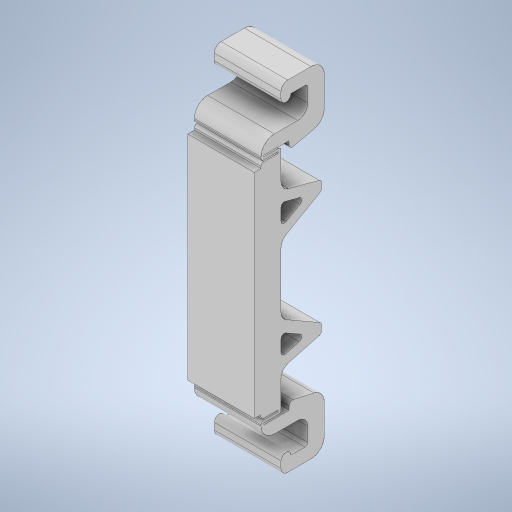
# Autodesk Inventor part: DIN-rail-mount
Saved by Autodesk Inventor 2023 (Build 270158030, 158C)
## iProperties
Created: 2024-03-20
Part Number: DIN-rail-mount
Material: Generic
Document SubType Name: Modeling
Designer: Imogen Heard
Density: 1 g/cm^3
Appearance: Default
Author: Imogen Heard
Autodesk Inventor part; units mm, degrees
ref_plane "YZ Plane" through (0, 0, 0) normal (1, 0, 0) x (0, 1, 0)
ref_plane "XZ Plane" through (0, 0, 0) normal (0, 1, 0) x (-1, 0, 0)
ref_plane "XY Plane" through (0, 0, 0) normal (0, 0, 1) x (1, 0, 0)
sketch "DIN-rail-clip-generic-V1.0" plane through (0, 0, 0) normal (0, 0, 1) x (1, 0, 0)
  line L0 (0, 40.9467) -> (3, 40.9467)
  line L1 (3, 40.9467) -> (3, 17.5)
  line L2 (3, 17.5) -> (0, 17.5)
  line L3 (0, 17.5) -> (0, 40.9467)
  line L4 (0, 35.1) -> (-0.3528, 35.269) construction
  line L5 (-0.3528, 35.269) -> (-1.1784, 35.269) construction
  line L6 (-1.1784, 35.269) -> (-1.277, 34.6657) construction
  line L7 (-1.277, 34.6657) -> (-0.9372, 34.5565) construction
  line L8 (-0.9372, 34.5565) -> (-2.5363, 34.2808) construction
  line L9 (-2.5363, 34.2808) -> (-3.3649, 34.5884) construction
  line L10 (-3.3649, 34.5884) -> (-4.7205, 35.8697) construction
  line L11 (-4.7205, 35.8697) -> (-5.1321, 37.4532) construction
  line L12 (-5.1321, 37.4532) -> (-5.1209, 40.8876) construction
  line L13 (-5.1209, 40.8876) -> (-4.7, 42.1113) construction
  line L14 (-4.7, 42.1113) -> (-3.9, 43.3113) construction
  line L15 (-3.9, 43.3113) -> (-2.1, 44.1113) construction
  line L16 (-2.1, 44.1113) -> (0, 43.5467) construction
  line L17 (0, 43.5467) -> (0.1036, 42.9467) construction
  line L18 (0.1036, 42.9467) -> (-0.2, 41.9467) construction
  line L19 (-0.2, 41.9467) -> (-1.1, 42.4004) construction
  line L20 (-1.1, 42.4004) -> (-2.3, 42.4379) construction
  spline S0 degree 4 poles (0, 35.1) (-0.3528, 35.269) (-1.1784, 35.269) (-1.277, 34.6657) (-0.9372, 34.5565) (-2.5363, 34.2808) (-3.3649, 34.5884) (-4.7205, 35.8697) (-5.1321, 37.4532) (-5.1209, 40.8876) (-4.7, 42.1113) (-3.9, 43.3113) (-2.1, 44.1113) (0, 43.5467) (0.1036, 42.9467) (-0.2, 41.9467) (-1.1, 42.4004) (-2.3, 42.4379) (-2.2829, 41.0379) (-1.7552, 41.1368) (0, 40.9467) knots 1 1 1 1 1 2 3 4 5 6 7 8 9 10 11 12 13 14 15 16 17 17.993985 17.993985 17.993985 17.993985 17.993985
  line L21 (0, 35.8905) -> (-0.7907, 36.0877) construction
  line L22 (-0.7907, 36.0877) -> (-1.1784, 36.0877) construction
  line L23 (-1.1784, 36.0877) -> (-2.2779, 36.5342) construction
  line L24 (-2.2779, 36.5342) -> (-2.7458, 36.6343) construction
  line L25 (-2.7458, 36.6343) -> (-3.471, 38.3527) construction
  line L26 (-3.471, 38.3527) -> (-2.7458, 40.1075) construction
  spline S1 degree 4 poles (0, 35.8905) (-0.7907, 36.0877) (-1.1784, 36.0877) (-2.2779, 36.5342) (-2.7458, 36.6343) (-3.471, 38.3527) (-2.7458, 40.1075) (-2.4429, 40.6075) (-0.7055, 40.4056) (0, 40.2568) knots 1 1 1 1 1 2 3 4 5 6 6.977977 6.977977 6.977977 6.977977 6.977977
  line L27 (-2.3, 42.4379) -> (-2.2829, 41.0379) construction
  line L28 (-2.2829, 41.0379) -> (-1.7552, 41.1368) construction
  line L29 (-1.7552, 41.1368) -> (0, 40.9467) construction
  line L30 (-2.7458, 40.1075) -> (-2.4429, 40.6075) construction
  line L31 (-2.4429, 40.6075) -> (-0.7055, 40.4056) construction
  line L32 (-0.7055, 40.4056) -> (0, 40.2568) construction
  line L33 (0, 36.6343) -> (-1.1784, 36.9758) construction
  line L34 (-1.1784, 36.9758) -> (-2.2101, 37.6402) construction
  line L35 (-2.2101, 37.6402) -> (-2.1452, 38.3006) construction
  line L36 (-2.1452, 38.3006) -> (-1.8076, 39.3817) construction
  line L37 (-1.8076, 39.3817) -> (-0.8778, 39.5886) construction
  line L38 (-0.8778, 39.5886) -> (0, 39.5886) construction
  spline S2 degree 4 poles (0, 36.6343) (-1.1784, 36.9758) (-2.2101, 37.6402) (-2.1452, 38.3006) (-1.8076, 39.3817) (-0.8778, 39.5886) (0, 39.5886) knots 1 1 1 1 1 2 3 4 4 4 4 4
  line L39 (-0.5144, 23.8721) -> (0, 22.0778) construction
  spline S3 degree 4 poles (0, 28.5164) (-0.0002, 28.5161) (-0.1764, 28.1682) (-0.5144, 27.8581) (-1.1668, 26.9412) (-3.3762, 27.1074) (-5.9868, 27.5396) (-6.4206, 26.5054) (-5.8606, 24.9054) (-2.8606, 24.6412) (-1.4606, 24.4656) (-0.5144, 23.8721) (0, 22.0778) knots 1 1 1 1 1 1.050464 1.110527 1.512977 1.739488 1.83789 2 2.236311 2.876473 3 3 3 3 3
  line L40 (-1.4606, 24.4656) -> (-0.5144, 23.8721) construction
  line L41 (-3.3762, 27.1074) -> (-5.9868, 27.5396) construction
  line L42 (-5.9868, 27.5396) -> (-6.4206, 26.5054) construction
  line L43 (-6.4206, 26.5054) -> (-5.8606, 24.9054) construction
  line L44 (-5.8606, 24.9054) -> (-2.8606, 24.6412) construction
  line L45 (-2.8606, 24.6412) -> (-1.4606, 24.4656) construction
  line L46 (0, 28.5164) -> (-0.1764, 28.1682) construction
  line L47 (-0.1764, 28.1682) -> (-0.5144, 27.8581) construction
  line L48 (-0.5144, 27.8581) -> (-1.1668, 26.9412) construction
  line L49 (-1.1668, 26.9412) -> (-3.3762, 27.1074) construction
  circle A0 centre (1, 40.9467) radius 0.7
  point P0 (0, 17.5)
  point P1 (-0.5, 35)
  point P2 (-1, 33.6)
  dimension "d63" = 3
  dimension "d68" = 23.4467
  dimension "d71" = 0.9373
  dimension "d73" = 0.269
  dimension "d74" = 0.3528
  dimension "d79" = 1.5363
  dimension "d85" = 0.7905
  dimension "d87" = 1.1784
  dimension "d88" = 0.7907
  dimension "d89" = 1.5835
  dimension "d90" = 5.1321
  dimension "d92" = 2.2779
  dimension "d93" = 2.7458
  dimension "d95" = 1.7184
  dimension "d96" = 0.7252
  dimension "d97" = 3.4344
  dimension "d99" = 1.2236
  dimension "d100" = 0.4209
  dimension "d101" = 1.2
  dimension "d102" = 0.8
  dimension "d103" = 1.8
  dimension "d104" = 0.8
  dimension "d105" = 2.6
  dimension "d106" = 0.1036
  dimension "d107" = 2
  dimension "d108" = 0.2
  dimension "d109" = 1
  dimension "d110" = 0.9
  dimension "d111" = 0.4536
  dimension "d112" = 1.2
  dimension "d113" = 1.4
  dimension "d114" = 0.0375
  dimension "d115" = 0.0171
  dimension "d116" = 0.5278
  dimension "d117" = 0.0989
  dimension "d118" = 0.69
  dimension "d119" = 0.6682
  dimension "d120" = 0.7055
  dimension "d121" = 0.5412
  dimension "d122" = 1.7374
  dimension "d123" = 0.2019
  dimension "d124" = 0.5
  dimension "d125" = 0.3029
  dimension "d126" = 1.1784
  dimension "d127" = 3.9709
  dimension "d128" = 0.6643
  dimension "d129" = 1.0316
  dimension "d130" = 0.6604
  dimension "d131" = 0.0649
  dimension "d132" = 1.8076
  dimension "d133" = 1.565
  dimension "d134" = 0.9298
  dimension "d136" = 0.7438
  dimension "d138" = 0.3482
  dimension "d139" = 0.3101
  dimension "d140" = 0.9169
  dimension "d141" = 2.2093
  dimension "d142" = 0.1662
  dimension "d143" = 0.1764
  dimension "d144" = 0.3381
  dimension "d145" = 0.6524
  dimension "d147" = 0.4338
  dimension "d148" = 1.6
  dimension "d149" = 0.56
  measures "d63" distance of the line from the sketch origin of L1
  measures "d68" distance between parallel lines of L2 L0
  measures "d73" vertical distance of L4.end point (-0.5, 35)
  measures "d79" horizontal distance of point (-1, 33.6) L8.end
  measures "d85" distance of L21.start L4.start
  measures "d89" vertical distance of L10.end L11.end
  measures "d95" vertical distance of L24.end L25.end
  measures "d96" horizontal distance of L25.end L24.end
  measures "d97" distance of L11.end L12.end
  measures "d99" vertical distance of L12.end L13.end
  measures "d100" horizontal distance of L13.end L12.end
  measures "d101" vertical distance of L14.end L13.end
  measures "d102" horizontal distance of L14.end L13.end
  measures "d103" horizontal distance of L15.end L14.end
  measures "d104" vertical distance of L14.end L15.end
  measures "d105" distance from line of L0 L16.end
  measures "d107" distance from line of L0 L17.end
  measures "d109" distance from line of L0 L18.end
  measures "d110" horizontal distance of L18.end L19.end
  measures "d111" vertical distance of L18.end L19.end
  measures "d112" horizontal distance of L19.end L20.end
  measures "d113" vertical distance of L27.end L20.end
  measures "d114" vertical distance of L20.end L19.end
  measures "d115" horizontal distance of L20.end L27.end
  measures "d116" horizontal distance of L27.end L28.end
  measures "d117" vertical distance of L27.end L28.end
  measures "d118" distance of L29.end L32.end
  measures "d119" distance of L38.end L32.end
  measures "d121" distance from line of L31.end L0
  measures "d122" horizontal distance of L30.end L31.end
  measures "d123" vertical distance of L30.end L31.end
  measures "d124" vertical distance of L26.end L30.end
  measures "d125" horizontal distance of L30.end L26.end
  measures "d127" distance from line of L0 L33.end
  measures "d128" vertical distance of L33.end L34.end
  measures "d129" horizontal distance of L33.end L34.end
  measures "d130" vertical distance of L35.end L34.end
  measures "d131" horizontal distance of L35.end L34.end
  measures "d133" distance from line of L36.end L0
  measures "d134" horizontal distance of L36.end L37.end
  measures "d136" distance of L21.start L33.start
  measures "d138" vertical distance of point (0, 28.516) L46.end
  measures "d139" vertical distance of L46.end L47.end
  measures "d140" vertical distance of L47.end L48.end
  measures "d141" horizontal distance of L49.end L48.end
  measures "d142" vertical distance of L48.end L49.end
  measures "d143" horizontal distance of L46.end point (0, 28.516)
  measures "d144" horizontal distance of L47.end L46.end
  measures "d145" horizontal distance of L47.end L48.end
  measures "d147" horizontal distance of L42.end L41.end
  measures "d148" vertical distance of L42.end L43.end
  measures "d149" horizontal distance of L43.end L42.end
sketch "Sketch1" plane through (0, 0, 0) normal (1, 0, 0) x (0, 1, 0)
  line L0 (5.8, -7.3) -> (29.2, -7.3)
  line L1 (29.2, -6.3) -> (5.8, -6.3)
  line L2 (32.2, -1) -> (35, -1)
  line L3 (35, -1) -> (35, 0)
  line L4 (35, 0) -> (32.2, 0)
  line L5 (-1817770.1114, -20.3632) -> (-1817770.1114, -1)
  line L6 (2.8, 0) -> (0, 0)
  line L7 (0, 0) -> (0, -1)
  line L8 (0, -1) -> (2.8, -1)
  line L9 (4.8, -2) -> (4.8, -5.3)
  arc A0 (32.2, -1) -> (31.2, -2) centre (32.2, -2) ccw
  arc A1 (29.2, -6.3) -> (30.2, -5.3) centre (29.2, -5.3) ccw
  arc A2 (4.8, -5.3) -> (5.8, -6.3) centre (5.8, -5.3) ccw
  arc A3 (3.8, -2) -> (2.8, -1) centre (2.8, -2) ccw
  arc A4 (4.8, -2) -> (2.8, 0) centre (2.8, -2) ccw
  arc A5 (3.8, -5.3) -> (5.8, -7.3) centre (5.8, -5.3) ccw
  line L10 (3.8, -2) -> (3.8, -5.3)
  arc A6 (32.2, 0) -> (30.2, -2) centre (32.2, -2) ccw
  arc A7 (29.2, -7.3) -> (31.2, -5.3) centre (29.2, -5.3) ccw
  line L11 (31.2, -2) -> (31.2, -5.3)
  line L12 (30.2, -2) -> (30.2, -5.3)
  line L13 (17.5, -4.8951) -> (17.5, -40.6352) construction
  point P0 (4.8, -3.65)
  dimension "d0" = 1
  dimension "d1" = 1
  dimension "d5" = 35
  dimension "d8" = 7.3
  dimension "d9" = 1
  dimension "d10" = 1
  dimension "d11" = 2
  dimension "d12" = 2
  dimension "d13" = 12.7
  dimension "d15" = 12.7
  dimension "d16" = 4.8
  dimension "d17" = 4.8
  dimension "d20" = 1
  dimension "d21" = 1
  dimension "d22" = 2
  constraints: 28 end point, 17 point on circle, 12 tangent, 8 centre point, 7 horizontal alignment, 4 equal radius, 4 parallel, 3 perpendicular, 2 horizontal, 2 vertical, 1 coincident, 1 midpoint, 1 point on line, 1 vertical alignment
  measures "d0" distance between parallel lines of L2 L4
  measures "d1" distance between parallel lines of L0 L1
  measures "d5" distance between parallel lines of L7 L3
  measures "d8" distance between parallel lines of L4 L0
  measures "d9" radius of A0
  measures "d10" radius of A1
  measures "d11" radius of A4
  measures "d12" radius of A6
  measures "d13" distance between parallel lines of L13 L12
  measures "d15" distance between parallel lines of L13 L9
  measures "d16" distance between parallel lines of L9 L7
  measures "d17" distance between parallel lines of L12 L3
  measures "d20" distance between parallel lines of L12 L11
  measures "d21" distance between parallel lines of L10 L9
  measures "d22" radius of A5
extrude "Extrusion5" add sketch "Sketch1" along normal blind 10
sketch "Sketch6" plane through (0, 0, 0) normal (1, 0, 0) x (0, 1, 0)
  arc A0 (3.8, -5.3) -> (5.8, -7.3) centre (5.8, -5.3) ccw projected
  line L0 (5.8, -7.3) -> (29.2, -7.3) projected
  arc A1 (29.2, -7.3) -> (31.2, -5.3) centre (29.2, -5.3) ccw projected
  line L1 (31.2, -5.3) -> (31.2, -2) projected
  arc A2 (32.2, -1) -> (31.2, -2) centre (32.2, -2) ccw projected
  line L2 (32.2, -1) -> (35, -1) projected
  line L3 (35, -1) -> (35, 0) projected
  line L4 (35, 0) -> (32.2, 0) projected
  arc A3 (32.2, 0) -> (30.2, -2) centre (32.2, -2) ccw projected
  line L5 (30.2, -2) -> (30.2, -5.3) projected
  arc A4 (29.2, -6.3) -> (30.2, -5.3) centre (29.2, -5.3) ccw projected
  line L6 (29.2, -6.3) -> (5.8, -6.3) projected
  arc A5 (4.8, -5.3) -> (5.8, -6.3) centre (5.8, -5.3) ccw projected
  line L7 (4.8, -5.3) -> (4.8, -2) projected
  arc A6 (4.8, -2) -> (2.8, 0) centre (2.8, -2) ccw projected
  line L8 (2.8, 0) -> (0, 0) projected
  line L9 (0, 0) -> (0, -1) projected
  line L10 (0, -1) -> (2.8, -1) projected
  arc A7 (3.8, -2) -> (2.8, -1) centre (2.8, -2) ccw projected
  line L11 (3.8, -2) -> (3.8, -5.3) projected
  line L12 (35, 0) -> (37, 0)
  line L13 (37, 0) -> (37, -2.5)
  line L14 (37, -6.5) -> (36.5978, -6.5)
  line L15 (35, -6.5) -> (35, 0)
  line L16 (38.5, -4) -> (40.6, -4)
  line L17 (43, -4) -> (43, -4.5)
  line L18 (41, -6.5) -> (37, -6.5)
  line L19 (37, -6.5) -> (37, -4)
  line L20 (43, -4) -> (41.117, -4)
  line L21 (35, -1.2) -> (34.4259, -1.2)
  line L22 (33.9382, -1.8104) -> (34.6472, -4.9417)
  line L23 (43, -4) -> (41, -4)
  line L24 (41, -3.6) -> (41, 0)
  line L25 (41, 0) -> (42, 0)
  line L26 (43, -1) -> (43, -4)
  line L27 (21.7121, 0) -> (17.5, 0)
  line L28 (17.5, 0) -> (17.5, 3)
  line L29 (34.8, 3) -> (35, 3)
  line L30 (37, 1) -> (37, 0)
  line L31 (35, -1) -> (35, 0) projected
  line L32 (35, 0) -> (34.8, 0)
  line L33 (34.8, 0.4) -> (34.8, 2.5)
  line L34 (34.9, 2.6) -> (34.9, 2.6)
  line L35 (35, 2.5) -> (35, 0)
  line L36 (34.4, 3) -> (34.2, 3)
  line L37 (34.2, 3) -> (34.2, 0.5)
  line L38 (34.3, 0.4) -> (34.3, 0.4)
  line L39 (34.4, 0.5) -> (34.4, 2.6)
  arc A8 (37, 1) -> (35, 3) centre (35, 1) ccw
  arc A9 (34.6472, -4.9417) -> (36.5978, -6.5) centre (36.5978, -4.5) ccw
  arc A10 (41, -6.5) -> (43, -4.5) centre (41, -4.5) ccw
  arc A11 (43, -1) -> (42, 0) centre (42, -1) ccw
  arc A12 (37, -2.5) -> (38.5, -4) centre (38.5, -2.5) ccw
  arc A13 (35, 2.5) -> (34.9, 2.6) centre (34.9, 2.5) ccw
  arc A14 (34.9, 2.6) -> (34.8, 2.5) centre (34.9, 2.5) ccw
  arc A15 (34.4, 0) -> (34.8, 0.4) centre (34.4, 0.4) ccw
  arc A16 (34.8, 3) -> (34.4, 2.6) centre (34.8, 2.6) ccw
  arc A17 (34.3, 0.4) -> (34.4, 0.5) centre (34.3, 0.5) ccw
  arc A18 (34.2, 0.5) -> (34.3, 0.4) centre (34.3, 0.5) ccw
  line L40 (33.8, 3) -> (17.5, 3)
  line L41 (17.5, 3) -> (17.5, 0)
  line L42 (30.2855, 0) -> (34.2, 0)
  line L43 (34.2, 0) -> (34.2, 2.6)
  arc A19 (34.2, 2.6) -> (33.8, 3) centre (33.8, 2.6) ccw
  circle A20 centre (41, -0.75) radius 0.75
  arc A21 (34.4259, -1.2) -> (33.9382, -1.8104) centre (34.4259, -1.7) ccw
  arc A22 (40.6, -4) -> (41, -3.6) centre (40.6, -3.6) ccw
  line L44 (17.5, 3) -> (33.5, 3)
  line L45 (33.5, 3) -> (33.5, 4)
  line L46 (33.5, 4) -> (17.5, 4)
  line L47 (17.5, 4) -> (17.5, 3)
  line L48 (28.8366, -1.1118) -> (27.5993, -5.7294)
  line L49 (29.2, -6.3) -> (5.8, -6.3) projected
  line L50 (25.9557, -5.85) -> (23.0112, -0.75)
  line L51 (27.1163, -6.1) -> (26.3887, -6.1)
  line L52 (27.4129, -0.6294) -> (26.857, -2.7041)
  line L53 (25.941, -2.8247) -> (24.7432, -0.75)
  arc A23 (30.2855, 0) -> (28.8366, -1.1118) centre (30.2855, -1.5) ccw
  arc A24 (23.0112, -0.75) -> (21.7121, 0) centre (21.7121, -1.5) ccw
  arc A25 (25.941, -2.8247) -> (26.857, -2.7041) centre (26.3741, -2.5747) ccw
  arc A26 (27.1163, -6.1) -> (27.5993, -5.7294) centre (27.1163, -5.6) ccw
  arc A27 (25.9557, -5.85) -> (26.3887, -6.1) centre (26.3887, -5.6) ccw
  line L54 (26.93, 0) -> (25.1762, 0)
  arc A28 (27.4129, -0.6294) -> (26.93, 0) centre (26.93, -0.5) ccw
  arc A29 (25.1762, 0) -> (24.7432, -0.75) centre (25.1762, -0.5) ccw
  point P0 (43, -6.5)
  point P1 (33.8, -1.2)
  point P2 (17.5, -6.3)
  point P3 (41, 0)
  point P4 (41, -1.5)
  point P5 (34.3, 0.4)
  point P6 (34.9, 2.6)
  point P7 (27.5, -6.1)
  point P8 (26.1, -6.1)
  point P9 (22.5782, 0)
  point P10 (27.5816, 0)
  point P11 (24.3102, 0)
  point P12 (35, -5.7029)
  point P13 (41, 0)
  dimension "d259" = 2.5
  dimension "d268" = 6
  dimension "d269" = 2
  dimension "d270" = 4
  dimension "d271" = 3
  dimension "d272" = 1.2
  dimension "d273" = 0.2
  dimension "d274" = 0.2
  dimension "d275" = 0.4
  dimension "d276" = 0.4
  dimension "d277" = 0.2
  dimension "d278" = 0.4
  dimension "d279" = 3
  dimension "d280" = 2
  dimension "d281" = 2
  dimension "d282" = 1
  dimension "d283" = 1.5
  dimension "d284" = 0.1
  dimension "d285" = 0.4
  dimension "d286" = 0.4
  dimension "d287" = 0.1
  dimension "d288" = 0.1
  dimension "d289" = 0.4
  dimension "d290" = 1.5
  dimension "d291" = 0.75
  dimension "d292" = 0.5
  dimension "d293" = 0.4
  dimension "d294" = 16
  dimension "d295" = 1
  dimension "d298" = 75
  dimension "d299" = 60
  dimension "d300" = 0.2
  dimension "d301" = 1.4
  dimension "d302" = 7.5
  dimension "d303" = 1.5
  dimension "d304" = 1.5
  dimension "d305" = 1.5
  dimension "d306" = 1.5
  dimension "d307" = 0.5
  dimension "d308" = 0.5
  constraints: 82 end point, 42 point on circle, 42 tangent, 35 point on line, 22 centre point, 17 parallel, 11 horizontal, 8 perpendicular, 6 equal radius, 1 horizontal alignment, 1 midpoint, 1 vertical alignment, 1 other
  measures "d259" distance between parallel lines of L18 L16
  measures "d268" distance between parallel lines of L13 L17
  measures "d269" distance between parallel lines of L24 L26
  measures "d270" distance between parallel lines of L25 L16
  measures "d271" distance between parallel lines of L29 L27
  measures "d272" distance from line of L15 point (33.8, -1.2)
  measures "d273" distance between parallel lines of L2 L21
  measures "d274" distance between parallel lines of L33 L35
  measures "d275" distance between parallel lines of L29 L34
  measures "d276" distance between parallel lines of L39 L33
  measures "d277" distance between parallel lines of L37 L39
  measures "d278" distance between parallel lines of L27 L38
  measures "d279" distance between parallel lines of L16 L2
  measures "d280" distance between parallel lines of L13 L15
  measures "d281" radius of A8
  measures "d282" radius of A11
  measures "d283" radius of A12
  measures "d284" radius of A13
  measures "d285" radius of A15
  measures "d286" radius of A16
  measures "d287" radius of A17
  measures "d288" radius of A18
  measures "d289" radius of A19
  measures "d290" diameter of A20
  measures "d291" distance from line of L25 A20.centre
  measures "d292" radius of A21
  measures "d293" radius of A22
  measures "d294" distance between parallel lines of L45 L47
  measures "d295" distance between parallel lines of L44 L46
  measures "d298" angle of L27 L48
  measures "d299" angle of L27 L50
  measures "d300" distance from line of L6 point (26.1, -6.1)
  measures "d301" distance of point (27.5, -6.1) point (26.1, -6.1)
  measures "d302" distance from line of L3 point (27.5, -6.1)
  measures "d303" distance between parallel lines of L50 L53
  measures "d304" distance between parallel lines of L48 L52
  measures "d305" radius of A23
  measures "d306" radius of A24
  measures "d307" radius of A25
  measures "d308" radius of A28
extrude "Extrusion6" add sketch "Sketch6" along normal blind 10 separate body contours L3 L12 L13 A12 L16 A22 L24 A20 L25 A11 L26 L17 A10 L18 L14 A9 L15 | L35 A13 A14 L33 A15 L4 L43 A18 A17 L39 A16 L29 A8 L30 L12 | L15 A9 L22 A21 L21 | L4 L42 A23 L48 A26 L51 A27 L50 A24 L27 L28 L40 A19 L37 L43 | A20 L24 | L24 A20 | L40 L47 L46 L45
mirror "Mirror2" about plane through (0, 17.5, 4) normal (0, -1, 0) of "Extrusion6" bodies 2
